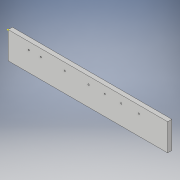
# Autodesk Inventor part: Bumper Middle
Saved by Autodesk Inventor 2018 (Build 220112000, 112)
## iProperties
Created: 2018-02-12
Part Number: Bumper Middle
Material: Generic
Document SubType Name: Modeling
Designer: kalra.rohan
Density: 1 g/cm^3
Appearance: Default
Author: kalra.rohan
Autodesk Inventor part; units mm, degrees
ref_plane "YZ Plane" through (0, 0, 0) normal (1, 0, 0) x (0, 1, 0)
ref_plane "XZ Plane" through (0, 0, 0) normal (0, 1, 0) x (-1, 0, 0)
ref_plane "XY Plane" through (0, 0, 0) normal (0, 0, 1) x (1, 0, 0)
sketch "Sketch1" plane through (0, 0, 0) normal (0, 0, 1) x (1, 0, 0)
  point P0 (0, 0)
sketch "Sketch2" plane through (0, 0, 0) normal (0, 0, 1) x (1, 0, 0)
  line L0 (0, 0) -> (855.98, 0)
  line L1 (855.98, 0) -> (855.98, -144.78)
  line L2 (855.98, -144.78) -> (0, -144.78)
  line L3 (0, -144.78) -> (0, 0)
  dimension "d0" = 855.98
  dimension "d1" = 144.78
  constraints: 8 end point, 2 parallel, 1 horizontal, 1 perpendicular
  measures "d0" distance between parallel lines of L1 L3
  measures "d1" distance between parallel lines of L0 L2
extrude "Extrusion1" add sketch "Sketch2" against normal blind 22.86
sketch "Sketch3" plane through (0, 0, 0) normal (0, 0, 1) x (1, 0, 0)
  circle A0 centre (702.2084, -39.7993) radius 3.918
  line L0 (855.98, 0) -> (855.98, -144.78)
  line L1 (855.98, -144.78) -> (0, -144.78)
  circle A1 centre (606.4377, -39.7993) radius 3.9179
  circle A2 centre (518.5029, -39.7993) radius 3.9179
  circle A3 centre (431.9651, -39.7993) radius 3.9179
  circle A4 centre (303.7332, -39.7993) radius 3.918
  circle A5 centre (175.5013, -39.7993) radius 3.918
  circle A6 centre (110.7948, -39.7993) radius 3.9179
  point P0 (0, 0)
  dimension "d4" = 153.7716
  dimension "d5" = 7.8359
  dimension "d6" = 104.9807
  dimension "d7" = 7.8359
  dimension "d8" = 87.9348
  dimension "d9" = 7.8359
  dimension "d10" = 87.9348
  dimension "d11" = 7.8359
  dimension "d12" = 86.5378
  dimension "d13" = 128.2319
  dimension "d14" = 7.8359
  dimension "d15" = 128.2319
  dimension "d16" = 7.8359
  dimension "d18" = 104.9807
  dimension "d19" = 104.9807
  dimension "d20" = 104.9807
  dimension "d21" = 104.9807
  dimension "d22" = 104.9807
  dimension "d23" = 104.9807
  constraints: 7 centre point
  measures "d4" distance from line of L0 A0.centre
  measures "d5" diameter of A0
  measures "d6" distance from line of A0.centre L1
  measures "d7" diameter of A1
  measures "d9" diameter of A2
  measures "d10" distance of A1.centre A2.centre
  measures "d11" diameter of A3
  measures "d12" distance of A2.centre A3.centre
  measures "d13" distance of A3.centre A4.centre
  measures "d14" diameter of A5
  measures "d15" distance of A4.centre A5.centre
  measures "d16" diameter of A6
  measures "d18" distance from line of A6.centre L1
  measures "d19" distance from line of A5.centre L1
  measures "d20" distance from line of A4.centre L1
  measures "d21" distance from line of A3.centre L1
  measures "d22" distance from line of A2.centre L1
  measures "d23" distance from line of L1 A1.centre
extrude "Extrusion2" cut sketch "Sketch3" against normal blind 304.8
body "Solid1"
